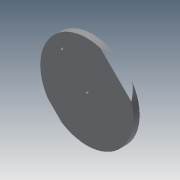
# Autodesk Inventor part: mainpulley
Saved by Autodesk Inventor 2015 (Build 190159000, 159)
## iProperties
Created: 2014-08-31
Part Number: mainpulley
Material: Generic
Document SubType Name: Modeling
Designer: shohei
Density: 1 g/cm^3
Appearance: Default
Mass: 1410.58 g
Surface Area: 1611.64 cm^2
Volume: 1410.58 cm^3
Author: shohei
Autodesk Inventor part; units mm, degrees
ref_plane "YZ Plane" through (0, 0, 0) normal (1, 0, 0) x (0, 1, 0)
ref_plane "XZ Plane" through (0, 0, 0) normal (0, 1, 0) x (-1, 0, 0)
ref_plane "XY Plane" through (0, 0, 0) normal (0, 0, 1) x (1, 0, 0)
sketch "Sketch1" plane through (0, 0, 0) normal (0, 1, 0) x (-1, 0, 0)
  circle A0 centre (0, 0) radius 150
  circle A1 centre (0, 0) radius 5
  circle A2 centre (81.3173, 81.3173) radius 5
  line L0 (210, 0) -> (-210, 0) projected
  line L1 (0, -210) -> (0, 210) projected
  dimension "d0" = 300
  dimension "d1" = 10
  dimension "d2" = 10
  dimension "d7" = 105
  constraints: 3 centre point, 2 coincident
  measures "d0" diameter of A0
  measures "d1" diameter of A1
  measures "d2" diameter of A2
extrude "Extrusion1" add sketch "Sketch1" along normal blind 20 contours L0 A1 L1 A0 | A0 L1 A1 L0 | L1 A1 L0 A0 | A0 L0 A1 L1
equation "\"d0\" = pD"
equation "\"d7\" = 0.35 * pD"
equation "\"pD\" = 300"
body "Solid1"
